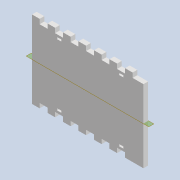
# Autodesk Inventor part: 00_Baseplate_Simmo_side7_v2
Saved by Autodesk Inventor 2022 (Build 260153000, 153)
## iProperties
Created: 2022-08-09
Part Number: 00_Baseplate_Simmo_side7_v2
Material: Generic
Document SubType Name: Modeling
Designer: wanghaoran
Density: 1 g/cm^3
Appearance: Default
Author: wanghaoran
Autodesk Inventor part; units mm, degrees
ref_plane "YZ Plane" through (0, 0, 0) normal (1, 0, 0) x (0, 1, 0)
ref_plane "XZ Plane" through (0, 0, 0) normal (0, 1, 0) x (-1, 0, 0)
ref_plane "XY Plane" through (0, 0, 0) normal (0, 0, 1) x (1, 0, 0)
sketch "Sketch1" plane through (0, 0, 0) normal (0, 0, 1) x (1, 0, 0)
  line L0 (-5, 0) -> (-5, 6) projected
  line L1 (138.8836, 0) -> (138.8836, 6) projected
  line L2 (138.8836, 6) -> (-5, 6)
  line L3 (-5, 6) -> (-5, -94)
  line L4 (-5, -94) -> (138.8836, -94)
  line L5 (138.8836, -94) -> (138.8836, 6)
  point P0 (0, 0)
  point P1 (-5, 6)
  dimension "d0" = 100
  constraints: 8 end point, 2 parallel, 1 horizontal, 1 perpendicular
  measures "d0" distance of L3.end L2.end
extrude "Extrusion1" add sketch "Sketch1" along normal blind 6
sketch "Sketch4" plane through (0, 0, 6) normal (0, 0, 1) x (1, 0, 0)
  line L0 (125, 0) -> (138.8836, 0) projected
  line L1 (125, 6) -> (125, 0) projected
  line L2 (138.8836, 0) -> (138.8836, 6) projected
  line L3 (125, 6) -> (138.8836, 6) projected
  line L4 (125, 0) -> (124.9, 0)
  line L5 (124.9, 0) -> (124.9, 6)
  line L6 (124.9, 6) -> (125, 6)
  line L7 (125, 6) -> (125, 0)
  point P0 (0, 0)
  dimension "d21" = 0.1
  dimension "d22" = 6
  constraints: 8 end point, 2 parallel, 1 horizontal, 1 perpendicular
  measures "d21" distance of L5.end L6.end
  measures "d22" distance of L4.end L5.end
extrude "Extrusion4" cut sketch "Sketch4" against normal through all
sketch "Sketch5" plane through (0, 0, 6) normal (0, 0, 1) x (1, 0, 0)
  line L0 (110, 0) -> (110, 6) projected
  line L1 (115, 0) -> (115, 6) projected
  line L2 (105, 6) -> (115, 6) projected
  line L3 (105, 6) -> (105, 0) projected
  line L4 (105, 0) -> (115, 0) projected
  line L5 (115, 0) -> (115.1, 0)
  line L6 (115.1, 0) -> (115.1, 6)
  line L7 (115.1, 6) -> (115, 6)
  line L8 (115, 6) -> (115, 0)
  line L9 (105, 0) -> (104.9, 0)
  line L10 (104.9, 0) -> (104.9, 6)
  line L11 (104.9, 6) -> (105, 6)
  line L12 (105, 6) -> (105, 0)
  point P0 (0, 0)
  dimension "d23" = 0.1
  dimension "d24" = 6
  dimension "d25" = 0.1
  dimension "d26" = 6
  constraints: 16 end point, 4 parallel, 2 horizontal, 2 perpendicular, 1 other
  measures "d23" distance of L7.end L6.end
  measures "d24" distance of L6.end L5.end
  measures "d25" distance of L10.end L11.end
  measures "d26" distance of L9.end L10.end
extrude "Extrusion5" cut sketch "Sketch5" against normal through all
pattern_linear "Rectangular Pattern2" count 6 spacing 20 along (-1, 0, 0) of "Extrusion5"
sketch "Sketch7" plane through (0, 0, 6) normal (0, 0, 1) x (1, 0, 0)
  line L0 (4.9, 6) -> (-5, 6) projected
  line L1 (-5, 6) -> (-4.9, 6)
  line L2 (-4.9, 6) -> (-4.9, 0)
  line L3 (-4.9, 0) -> (-5, 0)
  line L4 (-5, 0) -> (-5, 6)
  point P0 (0, 0)
  dimension "d27" = 0.1
  dimension "d28" = 6
  constraints: 8 end point, 2 parallel, 1 horizontal, 1 perpendicular
  measures "d27" distance of L2.end L3.end
  measures "d28" distance of L1.end L2.end
extrude "Extrusion6" cut sketch "Sketch7" against normal through all
ref_plane "Work Plane1" through (-5, -44, 0) normal (0, -1, 0) x (1, 0, 0)
mirror "Mirror1" about plane through (-5, -44, 0) normal (0, -1, 0) of "Extrusion5", "Rectangular Pattern2"
sketch "Sketch8" plane through (0, 0, 6) normal (0, 0, 1) x (1, 0, 0)
  line L0 (112.75, -5.4) -> (107.25, -5.4)
  line L1 (107.25, -5.4) -> (107.25, -3)
  line L2 (107.25, -3) -> (112.75, -3)
  line L3 (112.75, -3) -> (112.75, -5.4)
  line L4 (104.9, 0) -> (104.9, 6) projected
  line L5 (115.1, 0) -> (104.9, 0) projected
  point P0 (0, 0)
  dimension "d31" = 5.5
  dimension "d32" = 2.4
  dimension "d33" = 2.35
  dimension "d34" = 3
  constraints: 8 end point, 2 parallel, 1 horizontal, 1 perpendicular
  measures "d31" distance of L1.end L2.end
  measures "d32" distance of L0.end L1.end
  measures "d33" distance between parallel lines of L4 L1
  measures "d34" distance between parallel lines of L5 L2
extrude "Extrusion7" cut sketch "Sketch8" against normal through all
pattern_linear "Rectangular Pattern3" count 2 spacing 80 along (-1, 0, 0) of "Extrusion7"
ref_plane "Work Plane2" through (138.8836, -44, 0) normal (0, -1, 0) x (1, 0, 0)
mirror "Mirror2" about plane through (138.8836, -44, 0) normal (0, -1, 0) of "Extrusion7", "Rectangular Pattern3"
body "Solid1"
